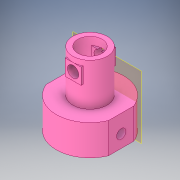
# Autodesk Inventor part: ActuatorCapPrecise
Saved by Autodesk Inventor 2017 (Build 210142000, 142)
## iProperties
Created: 2017-03-13
Part Number: ActuatorCapPrecise
Material: Generic
Document SubType Name: Modeling
Designer: Joseph
Density: 1 g/cm^3
Appearance: Pink
Author: Joseph
Autodesk Inventor part; units mm, degrees
ref_plane "YZ Plane" through (0, 0, 0) normal (1, 0, 0) x (0, 1, 0)
ref_plane "XZ Plane" through (0, 0, 0) normal (0, 1, 0) x (-1, 0, 0)
sketch "Sketch1" plane through (0, 0, 0) normal (0, 1, 0) x (-1, 0, 0)
  circle A0 centre (0, 0) radius 6.5
  dimension "d0" = 13
  constraints: 1 centre point, 1 coincident
  measures "d0" diameter of A0
extrude "Extrusion1" add sketch "Sketch1" along normal blind 14
sketch "Sketch2" plane through (0, 14, 0) normal (0, 1, 0) x (1, 0, 0)
  line L0 (3.3985, -3.1) -> (-3.3985, -3.1)
  line L1 (3.3985, 3.1) -> (-3.3985, 3.1)
  arc A0 (-3.3985, 3.1) -> (-3.3985, -3.1) centre (0, 0) ccw
  arc A1 (3.3985, -3.1) -> (3.3985, 3.1) centre (0, 0) ccw
  dimension "d3" = 4.6
  dimension "d4" = 4.6
  dimension "d7" = 6.2
  constraints: 4 end point, 4 point on circle, 2 centre point, 2 coincident, 2 horizontal, 1 parallel
  measures "d3" radius of A1
  measures "d4" radius of A0
  measures "d7" distance between parallel lines of L1 L0
extrude "Extrusion2" cut sketch "Sketch2" against normal blind 7.8
sketch "Sketch3" plane through (-3.3985, 14, -3.1) normal (0, 0, 1) x (1, 0, 0)
  circle A0 centre (3.5144, -3) radius 2.125
  line L0 (0, 0) -> (6.7971, 0) projected
  line L1 (3.5144, -3) -> (0.1159, -3)
  line L2 (3.5144, -3) -> (6.9129, -3)
  point P0 (3.3985, -14)
  dimension "d10" = 4.25
  dimension "d11" = 3
  constraints: 4 end point, 2 horizontal, 1 centre point, 1 collinear
  measures "d10" diameter of A0
  measures "d11" distance from line of L0 L1.start
extrude "Extrusion3" cut sketch "Sketch3" along normal mid plane 20
sketch "Sketch4" plane through (0, 0, 0) normal (0, -1, 0) x (1, 0, 0)
  circle A0 centre (0, 0) radius 12.7
  dimension "d14" = 25.4
  constraints: 1 centre point, 1 coincident
  measures "d14" diameter of A0
extrude "Extrusion4" add sketch "Sketch4" along normal blind 2
sketch "Sketch5" plane through (0, -2, 0) normal (0, -1, 0) x (1, 0, 0)
  circle A0 centre (0, 0) radius 4.8125
  circle A1 centre (0, 0) radius 12.7 projected
  line L0 (-11.7732, -4.7625) -> (11.7732, -4.7625)
  line L1 (11.7732, -4.7625) -> (11.7732, 4.7625)
  line L2 (11.7732, 4.7625) -> (-11.7732, 4.7625)
  line L3 (-11.7732, 4.7625) -> (-11.7732, -4.7625)
  line L4 (-11.7732, -4.7625) -> (11.7732, 4.7625) construction
  line L5 (11.7732, -4.7625) -> (-11.7732, 4.7625) construction
  arc A2 (11.7732, 4.7625) -> (-11.7732, 4.7625) centre (0, 0) ccw
  arc A3 (-11.7732, -4.7625) -> (11.7732, -4.7625) centre (0, 0) ccw
  line L6 (11.7732, 4.7625) -> (-11.7732, 4.7625)
  line L7 (-11.7732, -4.7625) -> (11.7732, -4.7625)
  dimension "d17" = 9.625
  dimension "d18" = 9.525
  constraints: 16 end point, 4 equal length, 4 point on circle, 3 centre point, 3 coincident, 2 midpoint, 1 horizontal, 1 perpendicular, 2 other
  measures "d17" diameter of A0
  measures "d18" distance of L2.end L0.start
extrude "Extrusion5" add sketch "Sketch5" along normal blind 9.525 contours A0 L0 L2 | A0 L2 L1 L0 | L2 A0 | A0 L2 A1 | L0 A1 A0 | A0 L0 | A0 L0 L3 L2
sketch "Sketch6" plane through (0, -11.525, 0) normal (0, -1, 0) x (1, 0, 0)
  circle A0 centre (0, 0) radius 4.8125
  dimension "d21" = 9.625
  constraints: 1 centre point, 1 coincident
  measures "d21" diameter of A0
extrude "Extrusion6" cut sketch "Sketch6" against normal blind 9.525
sketch "Sketch7" plane through (0, -2, 0) normal (0, -1, 0) x (1, 0, 0)
  line L0 (11.7732, -4.7625) -> (11.7732, 4.7625) projected
  line L1 (11.7732, 4.7625) -> (11.7732, -4.7625)
  line L2 (-11.7732, 4.7625) -> (-11.7732, -4.7625) projected
  line L3 (-11.7732, 4.7625) -> (-11.7732, -4.7625)
  arc A0 (11.7732, 4.7625) -> (-11.7732, 4.7625) centre (0, 0) ccw projected
  arc A1 (11.7732, -4.7625) -> (11.7732, 4.7625) centre (0, 0) ccw
  arc A2 (-11.7732, 4.7625) -> (-11.7732, -4.7625) centre (0, 0) ccw
  dimension "d24" = 12.7
  constraints: 4 end point, 4 point on circle, 2 centre point, 2 collinear, 1 concentric
  measures "d24" radius of A1
extrude "Extrusion7" cut sketch "Sketch7" against normal blind 9.525
sketch "Sketch8" plane through (11.7732, -11.525, 4.7625) normal (1, 0, 0) x (0, 0, -1)
  circle A0 centre (4.7625, 4.7625) radius 1.7526
  line L0 (4.7625, 4.7625) -> (4.7625, 11.525)
  line L1 (-1.7375, 11.525) -> (11.2625, 11.525) projected
  line L2 (9.525, 0) -> (0, 0) projected
  dimension "d27" = 3.5052
  dimension "d28" = 4.7625
  constraints: 2 end point, 1 centre point, 1 perpendicular
  measures "d27" diameter of A0
  measures "d28" distance from line of L0.start L2
extrude "Extrusion8" cut sketch "Sketch8" against normal blind 25.4
ref_plane "Work Plane1" through (0, 0, -6.5) normal (0, 0, 1) x (1, 0, 0)
sketch "Sketch9" plane through (0, 0, -6.5) normal (0, 0, 1) x (1, 0, 0)
  line L0 (-2.0091, 8.875) -> (2.2409, 8.875)
  line L1 (2.2409, 8.875) -> (2.2409, 13.125)
  line L2 (2.2409, 13.125) -> (-2.0091, 13.125)
  line L3 (-2.0091, 13.125) -> (-2.0091, 8.875)
  line L4 (-2.0091, 8.875) -> (2.2409, 13.125) construction
  line L5 (2.2409, 8.875) -> (-2.0091, 13.125) construction
  circle A0 centre (0.1159, 11) radius 2.125 projected
  line L6 (6.5, 14) -> (-6.5, 14) projected
  line L7 (-2.8841, 8) -> (3.1159, 8)
  line L8 (3.1159, 8) -> (3.1159, 14)
  line L9 (3.1159, 14) -> (-2.8841, 14)
  line L10 (-2.8841, 14) -> (-2.8841, 8)
  line L11 (-2.8841, 8) -> (3.1159, 14) construction
  line L12 (3.1159, 8) -> (-2.8841, 14) construction
  arc A1 (0.1159, 8.875) -> (2.2409, 11) centre (0.1159, 11) ccw
  arc A2 (-2.0091, 11) -> (0.1159, 8.875) centre (0.1159, 11) ccw
  arc A3 (0.1159, 13.125) -> (-2.0091, 11) centre (0.1159, 11) ccw
  arc A4 (2.2409, 11) -> (0.1159, 13.125) centre (0.1159, 11) ccw
  point P0 (0, 0)
  point P1 (0.1159, 11)
  constraints: 24 end point, 8 point on circle, 5 midpoint, 4 centre point, 4 coincident, 4 horizontal, 4 parallel, 3 perpendicular, 2 vertical, 1 horizontal alignment, 1 point on line, 1 other
extrude "Extrusion9" add sketch "Sketch9" along normal blind 13 contours L3 A0 L0 | A0 L1 L0 | L3 L2 A0 | A0 L2 L1 | L8 L7 L10 L6
sketch "Sketch10" plane through (0, 14, 0) normal (0, 1, 0) x (1, 0, 0)
  circle A0 centre (0, 0) radius 4.6
  constraints: 1 centre point, 1 coincident
extrude "Extrusion10" cut sketch "Sketch10" against normal up to surface (14 mm away)
sketch "Sketch11" plane through (0, -11.525, 0) normal (0, -1, 0) x (1, 0, 0)
  circle A0 centre (0, 0) radius 5.334
  dimension "d36" = 10.668
  constraints: 1 centre point, 1 coincident
  measures "d36" diameter of A0
extrude "Extrusion11" cut sketch "Sketch11" against normal up to surface (9.525 mm away)
sketch "Sketch12" plane through (0, 14, 0) normal (0, 1, 0) x (1, 0, 0)
  circle A0 centre (0, 0) radius 6.5
  circle A1 centre (0, 0) radius 4.6
  constraints: 2 centre point, 2 coincident
extrude "Extrusion12" add sketch "Sketch12" along normal blind 2
sketch "Sketch13" plane through (0, 0, 0) normal (0, 1, 0) x (1, 0, 0)
  line L0 (-2.985, 3.5) -> (2.985, 3.5)
  circle A0 centre (0, 0) radius 4.6 projected
  line L1 (-2.985, -3.5) -> (2.985, -3.5)
  arc A1 (2.985, 3.5) -> (-2.985, 3.5) centre (0, 0.0834) ccw
  arc A2 (2.985, -3.5) -> (-2.985, -3.5) centre (0, 0) ccw
  arc A3 (2.985, 3.5) -> (-2.985, 3.5) centre (0, 0.0834) ccw
  dimension "d41" = 7
  constraints: 11 point on circle, 4 end point, 3 centre point, 2 parallel, 1 concentric, 1 horizontal
  measures "d41" distance between parallel lines of L1 L0
extrude "Extrusion13" add sketch "Sketch13" along normal up to surface (16 mm away) contours A0 L0 | A1 A0 | L1 A0
sketch "Sketch14" plane through (0, 16, 0) normal (0, 1, 0) x (1, 0, 0)
  circle A0 centre (0, 0) radius 4.6
  constraints: 1 centre point, 1 coincident
extrude "Extrusion14" cut sketch "Sketch14" against normal blind 3
sketch "Sketch15" plane through (0, 0, 6.5) normal (0, 0, 1) x (1, 0, 0)
  circle A0 centre (0.1159, 11) radius 2.125 projected
  line L0 (-2.0091, 11) -> (2.2409, 11)
  line L1 (0.1159, 8.875) -> (0.1159, 13.125)
  circle A1 centre (0.1159, 11) radius 2.125
  point P0 (0, 0)
  constraints: 4 end point, 4 point on circle, 1 centre point, 1 coincident, 1 concentric, 1 horizontal, 1 perpendicular
extrude "Extrusion15" cut sketch "Sketch15" against normal up to surface (13 mm away)
body "Solid1"
